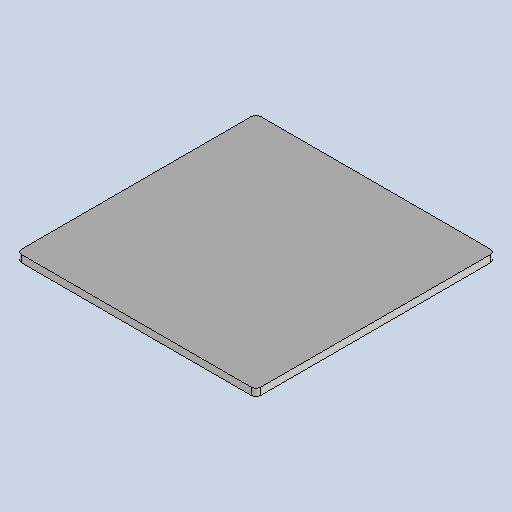
# Autodesk Inventor part: PNS 765 FDS 1200 CUP 1
Saved by Autodesk Inventor 2025.3 (Build 293356030, 356C)
## iProperties
Created: 2025-06-24
Part Number: PNS 765 FDS 1200 CUP 1
Material: Stainless Steel
Document SubType Name: Sheet Metal
Designer: user
Mass: 239.918 g
Surface Area: 211.828 cm^2
Volume: 29.9897 cm^3
Density: 8 g/cm^3
Flat Pattern Width: 10 cm
Flat Pattern Length: 10 cm
Flat Pattern Area: 100 cm^2
Sheet Metal Rule: AISI304 2mm Die16
Sheet Metal Width: 100,000 mm
Sheet Metal Length: 100,000 mm
Sheet Metal Area: 10000,000 mm^2
Appearance: Default
Author: user
Autodesk Inventor part; units mm, degrees
ref_plane "YZ Plane" through (0, 0, 0) normal (1, 0, 0) x (0, 1, 0)
ref_plane "XZ Plane" through (0, 0, 0) normal (0, 1, 0) x (-1, 0, 0)
ref_plane "XY Plane" through (0, 0, 0) normal (0, 0, 1) x (1, 0, 0)
sketch "Sketch1" plane through (0, 0, 0) normal (0, 0, 1) x (1, 0, 0)
  line L0 (-50, -50) -> (50, -50)
  line L1 (50, -50) -> (50, 50)
  line L2 (50, 50) -> (-50, 50)
  line L3 (-50, 50) -> (-50, -50)
  line L4 (-50, -50) -> (50, 50) construction
  line L5 (50, -50) -> (-50, 50) construction
  point P0 (0, 0)
  dimension "d154" = 100
  dimension "d155" = 100
  measures "d154" distance of L1.end L2.end
  measures "d155" distance of L0.end L1.end
extrude "Plate5" add sketch "Sketch1" along normal blind 3
fillet "Corner Round1" radius 2 4 edges at (50, 50, 1.5) (-50, 50, 1.5) (-50, -50, 1.5) (50, -50, 1.5)
body "Solid3"
